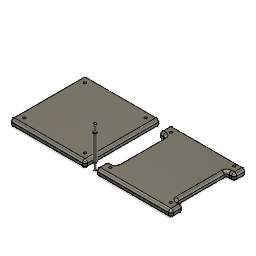
DKVprogetto_1.3 v1 (Autodesk Fusion 360 design; units mm, degrees)
Autodesk Fusion 360 part; units mm, degrees
sketch "Sketch1" plane through (0, 0, 0) normal (0, 1, 0) x (1, 0, 0)
  line L0 (-40, -10) -> (100, -10)
  line L1 (-40, 140) -> (100, 140)
  line L2 (-45, -5) -> (-45, 10)
  line L3 (-45, 135) -> (-45, 120)
  line L4 (-40, 15) -> (-35, 15)
  line L5 (-30, 20) -> (-30, 110)
  line L6 (100, 15) -> (95, 15)
  line L7 (90, 20) -> (90, 110)
  line L8 (-40, 115) -> (-35, 115)
  line L9 (-45, 120) -> (-45, 135)
  line L10 (105, 135) -> (105, 120)
  line L11 (100, 115) -> (95, 115)
  line L12 (-45, -5) -> (-45, 10)
  line L13 (105, -5) -> (105, 10)
  arc A0 (-40, 15) -> (-45, 10) centre (-40, 10) ccw
  arc A1 (-35, 15) -> (-30, 20) centre (-35, 20) ccw
  arc A2 (-45, -5) -> (-40, -10) centre (-40, -5) ccw
  arc A3 (90, 20) -> (95, 15) centre (95, 20) ccw
  arc A4 (105, 10) -> (100, 15) centre (100, 10) ccw
  arc A5 (100, -10) -> (105, -5) centre (100, -5) ccw
  arc A6 (95, 115) -> (90, 110) centre (95, 110) ccw
  arc A7 (100, 115) -> (105, 120) centre (100, 120) ccw
  arc A8 (105, 135) -> (100, 140) centre (100, 135) ccw
  arc A9 (-40, 140) -> (-45, 135) centre (-40, 135) ccw
  arc A10 (-45, 120) -> (-40, 115) centre (-40, 120) ccw
  arc A11 (-30, 110) -> (-35, 115) centre (-35, 110) ccw
  circle A12 centre (-30, 5) radius 2.5
  circle A13 centre (90, 5) radius 2.5
  circle A14 centre (-30, 125) radius 2.5
  circle A15 centre (90, 130) radius 2.5
  line L14 (-65, 135) -> (-65, -5)
  line L15 (-70, -10) -> (-210, -10)
  line L16 (-215, -5) -> (-215, 135)
  line L17 (-210, 140) -> (-70, 140)
  arc A16 (-65, 135) -> (-70, 140) centre (-70, 135) ccw
  arc A17 (-70, -10) -> (-65, -5) centre (-70, -5) ccw
  arc A18 (-210, 140) -> (-215, 135) centre (-210, 135) ccw
  arc A19 (-215, -5) -> (-210, -10) centre (-210, -5) ccw
  circle A20 centre (-80, 5) radius 2.5
  circle A21 centre (-80, 125) radius 2.5
  circle A22 centre (-200, 125) radius 2.5
  circle A23 centre (-200, 5) radius 2.5
  dimension "d23" = 5
  dimension "d24" = 5
  dimension "d25" = 5
  dimension "d26" = 5
  dimension "d27" = 150
  dimension "d28" = 5
  dimension "d29" = 5
  dimension "d30" = 5
  dimension "d31" = 5
  dimension "d32" = 5
  dimension "d33" = 5
  dimension "d34" = 5
  dimension "d35" = 5
  measures "d23" diameter of A12
  measures "d24" diameter of A13
  measures "d25" diameter of A14
  measures "d26" diameter of A15
  measures "d28" radius of A16
  measures "d29" radius of A17
  measures "d30" radius of A18
  measures "d31" radius of A19
  measures "d32" diameter of A20
  measures "d33" diameter of A21
  measures "d34" diameter of A22
  measures "d35" diameter of A23
extrude "Extrude1" add sketch "Sketch1" along normal blind 15 makes body 1 at (50, 0, -50) makes body 2 at (-120.5644, 0, -45.6131)
sketch "Sketch2" plane through (0, 0, 0) normal (0, 1, 0) x (1, 0, 0)
fillet "Fillet1" radius 5 8 edges at (-65, 15, -65) (-66.4645, 15, -138.5355) (-140, 15, -140) (-213.5355, 15, -138.5355) (-215, 15, -65) (-213.5355, 15, 8.5355) (-140, 15, 10) (-66.4645, 15, 8.5355) on bodies 2
fillet "Fillet2" radius 5 8 edges at (-213.5355, 0, 8.5355) (-215, 0, -65) (-213.5355, 0, -138.5355) (-140, 0, -140) (-66.4645, 0, -138.5355) (-65, 0, -65) (-66.4645, 0, 8.5355) (-140, 0, 10) on bodies 2
fillet "Fillet3" radius 5 24 edges at (105, 15, -2.5) (103.5355, 15, -13.5355) (97.5, 15, -15) (91.4645, 15, -16.4645) (90, 15, -65) (91.4645, 15, -113.5355) (97.5, 15, -115) (103.5355, 15, -116.4645) (105, 15, -127.5) (103.5355, 15, -138.5355) (30, 15, -140) (-43.5355, 15, -138.5355) (-45, 15, -127.5) (-43.5355, 15, -116.4645) (-37.5, 15, -115) (-31.4645, 15, -113.5355) (-30, 15, -65) (-31.4645, 15, -16.4645) (-37.5, 15, -15) (-43.5355, 15, -13.5355) (-45, 15, -2.5) (-43.5355, 15, 8.5355) (30, 15, 10) (103.5355, 15, 8.5355) on bodies 1
fillet "Fillet4" radius 5 24 edges at (105, 0, -2.5) (103.5355, 0, -13.5355) (97.5, 0, -15) (91.4645, 0, -16.4645) (90, 0, -65) (91.4645, 0, -113.5355) (97.5, 0, -115) (103.5355, 0, -116.4645) (105, 0, -127.5) (103.5355, 0, -138.5355) (30, 0, -140) (-43.5355, 0, -138.5355) (-45, 0, -127.5) (-43.5355, 0, -116.4645) (-37.5, 0, -115) (-31.4645, 0, -113.5355) (-30, 0, -65) (-31.4645, 0, -16.4645) (-37.5, 0, -15) (-43.5355, 0, -13.5355) (-45, 0, -2.5) (-43.5355, 0, 8.5355) (30, 0, 10) (103.5355, 0, 8.5355) on bodies 1
sketch "Sketch3" plane through (0, 0, 0) normal (0, 1, 0) x (1, 0, 0)
sketch "Sketch4" plane through (0, 0, 0) normal (0, 0, 1) x (1, 0, 0)
  line L0 (-55, 0) -> (-52.5, 0)
  line L1 (-52.5, 0) -> (-52.5, 15)
  line L2 (-52.5, 15) -> (-51.5, 15)
  line L3 (-51.5, 15) -> (-51.5, 65)
  line L4 (-51.5, 65) -> (-52.5, 65)
  line L5 (-52.5, 65) -> (-52.5, 80)
  line L6 (-52.5, 80) -> (-55, 80)
  line L7 (-55, 80) -> (-55, 0)
  dimension "d43" = 2.5
  dimension "d44" = 1
sketch "Sketch5" plane through (0, 0, 0) normal (0, 1, 0) x (1, 0, 0)
  circle A0 centre (-55, 0) radius 2.5
sweep "Sweep1" add profiles "Sketch4" path "Sketch5" along A0 section 1 separate body makes body 3
